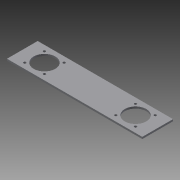
# Autodesk Inventor part: panel
Saved by Autodesk Inventor 2015 (Build 190159000, 159)
## iProperties
Created: 2014-08-06
Part Number: panel
Material: Generic
Document SubType Name: Modeling
Designer: Patrick Camilleri
Density: 1 g/cm^3
Appearance: Default
Author: Patrick Camilleri
Autodesk Inventor part; units mm, degrees
ref_plane "YZ Plane" through (0, 0, 0) normal (1, 0, 0) x (0, 1, 0)
ref_plane "XZ Plane" through (0, 0, 0) normal (0, 1, 0) x (-1, 0, 0)
ref_plane "XY Plane" through (0, 0, 0) normal (0, 0, 1) x (1, 0, 0)
sketch "Sketch1" plane through (0, 0, 0) normal (0, 0, 1) x (1, 0, 0)
  line L0 (-110, 25) -> (110, 25)
  line L1 (110, 25) -> (110, -25)
  line L2 (110, -25) -> (-110, -25)
  line L3 (-110, -25) -> (-110, 25)
  line L4 (-110, 25) -> (110, -25) construction
  line L5 (110, 25) -> (-110, -25) construction
  point P0 (0, 0)
  dimension "d0" = 220
  dimension "d1" = 50
  constraints: 12 end point, 2 midpoint, 2 parallel, 1 horizontal, 1 perpendicular
  measures "d0" distance of L1.end L2.end
  measures "d1" distance of L0.end L1.end
extrude "Extrusion1" add sketch "Sketch1" along normal blind 3
sketch "Sketch2" plane through (0, 0, 3) normal (0, 0, 1) x (1, 0, 0)
  line L0 (110, 25) -> (-110, 25) projected
  line L1 (-110, 25) -> (-110, -25) projected
  line L2 (0, -33.6991) -> (0, 32.9182) construction
  point P0 (0, 0)
  point P1 (-90, 16)
  point P2 (-58, 16)
  point P3 (-90, -16)
  point P4 (-58, -16)
  point P5 (90, 16)
  point P6 (58, 16)
  point P7 (90, -16)
  point P8 (58, -16)
  dimension "d8" = 32
  dimension "d11" = 32
  dimension "d14" = 9
  dimension "d15" = 20
  constraints: 4 symmetric about line, 2 end point, 2 vertical, 1 horizontal, 3 other
  measures "d8" distance of point (-90, 16) point (-58, 16)
  measures "d11" distance of point (-90, 16) point (-90, -16)
  measures "d14" distance from line of L0 point (-90, 16)
  measures "d15" distance from line of L1 point (-90, 16)
hole "Hole1" at (-90, 16, 3) at (-58, 16, 3) at (-90, -16, 3) at (-58, -16, 3) at (90, -16, 3) at (58, -16, 3) at (58, 16, 3) at (90, 16, 3) direction (0, 0, -1) diameter 4 end through all
sketch "Sketch3" plane through (0, 0, 3) normal (0, 0, 1) x (1, 0, 0)
  circle A0 centre (-90, -16) radius 2 projected
  circle A1 centre (-90, 16) radius 2 projected
  circle A2 centre (-58, 16) radius 2 projected
  circle A3 centre (-58, -16) radius 2 projected
  line L0 (-90, 16) -> (-58, -16) construction
  line L1 (-90, -16) -> (-58, 16) construction
  circle A4 centre (-74, 0) radius 17.5
  line L2 (0, -34.28) -> (0, 28.6476) construction
  circle A5 centre (74, 0) radius 17.5
  point P0 (0, 0)
  dimension "d23" = 35
  constraints: 6 end point, 2 centre point, 1 midpoint, 1 symmetric about line, 1 vertical, 1 other
  measures "d23" diameter of A4
extrude "Extrusion2" cut sketch "Sketch3" against normal blind 3 contours A4 | A5
body "Solid1"
